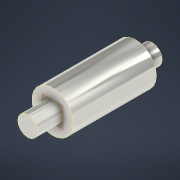
# Autodesk Inventor part: M2
Saved by Autodesk Inventor 2022 (Build 260153000, 153)
## iProperties
Created: 2022-01-10
Part Number: M2
Material: Silver
Document SubType Name: Modeling
Designer: student
Density: 10.49 g/cm^3
Appearance: Silver
Author: student
Autodesk Inventor part; units mm, degrees
ref_plane "YZ Plane" through (0, 0, 0) normal (1, 0, 0) x (0, 1, 0)
ref_plane "XZ Plane" through (0, 0, 0) normal (0, 1, 0) x (-1, 0, 0)
ref_plane "XY Plane" through (0, 0, 0) normal (0, 0, 1) x (1, 0, 0)
sketch "Sketch1" plane through (0, 0, 0) normal (0, 0, 1) x (1, 0, 0)
  circle A0 centre (-2.0967, 1.4241) radius 1.2
  point P0 (0, 0)
  dimension "d0" = 2.4
  constraints: 1 centre point
  measures "d0" diameter of A0
extrude "Extrusion1" add sketch "Sketch1" along normal blind 15
ref_plane "Work Plane1" through (-2.0967, 1.4241, 12) normal (0, 0, 1) x (1, 0, 0)
sketch "Sketch3" plane through (-2.0967, 1.4241, 12) normal (0, 0, 1) x (1, 0, 0)
  circle A0 centre (0, 0) radius 1.2 projected
  circle A1 centre (0, 0) radius 1.2 projected
  circle A2 centre (0, 0) radius 2.5
  point P0 (2.0967, -1.4241)
  dimension "d4" = 5
  constraints: 1 centre point, 1 coincident
  measures "d4" diameter of A2
extrude "Extrusion2" add sketch "Sketch3" against normal blind 10
body "Solid1"
